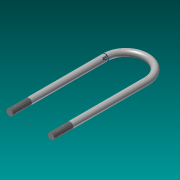
# Autodesk Inventor part: U BOLT
Saved by Autodesk Inventor 2014 SP2 (Build 180246200, 246)
## iProperties
Created: 2019-07-17
Part Number: U BOLT
Material: Steel, Mild
Document SubType Name: Modeling
Designer: USER PC
Density: 7.86 g/cm^3
Appearance: Steel
Mass: 248.227 g
Surface Area: 134.178 cm^2
Volume: 31.581 cm^3
Author: USER PC
Autodesk Inventor part; units mm, degrees
sketch "Sketch1" plane through (0, 0, 0) normal (0, 0, 1) x (1, 0, 0)
  line L0 (0, 0) -> (0, 150)
  line L1 (65, 0) -> (65, 150)
  line L2 (0, 0) -> (65, 0)
  arc A0 (65, 150) -> (0, 150) centre (32.5, 150) ccw
  line L3 (65, 0) -> (65, 30)
  line L4 (0, 0) -> (0, 30)
  line L5 (0, 150) -> (65, 150)
  dimension "d40" = 150
  dimension "d51" = 65
  dimension "d55" = 65
  dimension "d56" = 30
  dimension "d57" = 30
  constraints: 12 end point, 2 point on circle, 2 point on line, 1 centre point, 1 perpendicular, 1 vertical
  measures "d40" distance of L1.end L1.start
  measures "d51" distance of L0.start L1.start
  measures "d55" diameter of A0
  measures "d56" distance of L1.start L3.end
  measures "d57" distance of L0.start L4.end
ref_plane "Work Plane1" through (0, 150, 0) normal (0, 1, 0) x (-1, 0, 0)
sketch "Sketch2" plane through (0, 150, 0) normal (0, 1, 0) x (-1, 0, 0)
  circle A0 centre (0, 0) radius 5
  dimension "d2" = 10
  constraints: 1 centre point, 1 coincident
  measures "d2" diameter of A0
ref_plane "Work Plane2" through (65, 150, 0) normal (0, 1, 0) x (-1, 0, 0)
sketch "Sketch3" plane through (65, 150, 0) normal (0, 1, 0) x (-1, 0, 0)
  circle A0 centre (0, 0) radius 5
  point P0 (65, 0)
  dimension "d3" = 10
  constraints: 1 centre point
  measures "d3" diameter of A0
ref_plane "Work Plane3" through (0, 0, 0) normal (0, 1, 0) x (-1, 0, 0)
sketch "Sketch4" plane through (0, 0, 0) normal (0, 1, 0) x (-1, 0, 0)
  circle A0 centre (0, 0) radius 5
  dimension "d4" = 10
  constraints: 1 centre point, 1 coincident
  measures "d4" diameter of A0
ref_plane "Work Plane4" through (65, 0, 0) normal (0, 1, 0) x (-1, 0, 0)
sketch "Sketch5" plane through (65, 0, 0) normal (0, 1, 0) x (-1, 0, 0)
  circle A0 centre (0, 0) radius 5
  point P0 (65, 0)
  dimension "d5" = 10
  constraints: 1 centre point
  measures "d5" diameter of A0
ref_plane "Work Plane6" through (30, 0, 0) normal (1, 0, 0) x (0, 1, 0)
sketch "Sketch6" plane through (30, 0, 0) normal (1, 0, 0) x (0, 1, 0)
  point P0 (0, 0)
sketch "Sketch7" plane through (30, 0, 0) normal (1, 0, 0) x (0, 1, 0)
  point P0 (0, 0)
sketch "Sketch11" plane through (30, 0, 0) normal (1, 0, 0) x (0, 1, 0)
  point P0 (0, 0)
sketch "Sketch13" plane through (30, 0, 0) normal (1, 0, 0) x (0, 1, 0)
  point P0 (0, 0)
ref_plane "Work Plane10" through (0, 30, 0) normal (0, 1, 0) x (-1, 0, 0)
ref_plane "Work Plane13" through (65, 30, 0) normal (0, 1, 0) x (-1, 0, 0)
sketch "Sketch17" plane through (65, 30, 0) normal (0, 1, 0) x (-1, 0, 0)
  circle A0 centre (0, 0) radius 5
  point P0 (65, 0)
  dimension "d81" = 10
  constraints: 1 centre point
  measures "d81" diameter of A0
sketch "Sketch18" plane through (0, 30, 0) normal (0, 1, 0) x (-1, 0, 0)
  circle A0 centre (0, 0) radius 5
  dimension "d82" = 10
  constraints: 1 centre point, 1 coincident
  measures "d82" diameter of A0
loft "Loft10" add profiles "Sketch5", "Sketch17"
loft "Loft11" add profiles "Sketch4", "Sketch18"
thread "Thread3" size "M10x1.5" class "6g" standard "ANSI Metric M Profile" full length
thread "Thread4" size "M10x1.5" class "6g" standard "ANSI Metric M Profile" full length
extrude "Extrusion3" add sketch "Sketch2" against normal blind 120 separate body
extrude "Extrusion4" add sketch "Sketch3" against normal blind 120 separate body
sweep "Sweep3" add profiles "Sketch2" path "Sketch1" separate body path curves A0
body "Solid6"
body "Solid7"
body "Solid8"
body "Solid9"
